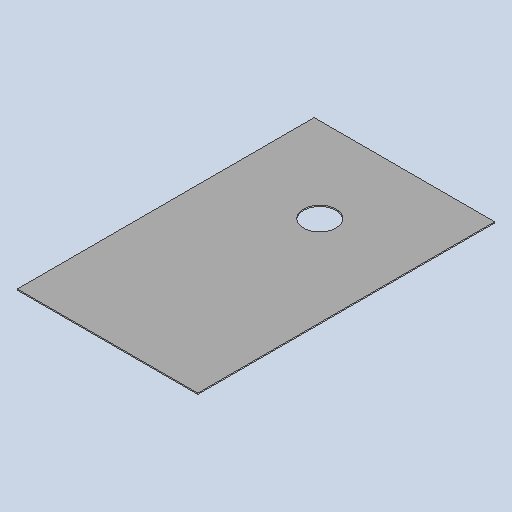
# Autodesk Inventor part: TRM 011 bottom main
Saved by Autodesk Inventor 2025 (Build 290162010, 162A)
## iProperties
Created: 2024-08-07
Part Number: TRM 011 bottom main
Material: AISI 304
Document SubType Name: Sheet Metal
Designer: pokla
Density: 8.02768 g/cm^3
Flat Pattern Width: 80.6 cm
Flat Pattern Length: 49 cm
Flat Pattern Area: 3949.4 cm^2
Sheet Metal Rule: AISI304 2mm Die16
Sheet Metal Width: 806.000 mm
Sheet Metal Length: 490.000 mm
Sheet Metal Area: 394940.000 mm^2
Appearance: Default
Stock Number: ТРМ 011 дно основное
Mass: 9361.53 g
Surface Area: 7860.53 cm^2
Volume: 1166.16 cm^3
Author: pokla
Autodesk Inventor part; units mm, degrees
ref_plane "YZ Plane" through (0, 0, 0) normal (1, 0, 0) x (0, 1, 0)
ref_plane "XZ Plane" through (0, 0, 0) normal (0, 1, 0) x (-1, 0, 0)
ref_plane "XY Plane" through (0, 0, 0) normal (0, 0, 1) x (1, 0, 0)
sketch "Sketch1" plane through (0, 0, 0) normal (0, 0, 1) x (1, 0, 0)
  line L0 (-245, -403) -> (245, -403)
  line L1 (245, -403) -> (245, 403)
  line L2 (245, 403) -> (-245, 403)
  line L3 (-245, 403) -> (-245, -403)
  line L4 (-245, -403) -> (245, 403) construction
  line L5 (245, -403) -> (-245, 403) construction
  point P0 (0, 0)
  dimension "d0" = 490
  dimension "d1" = 806
  measures "d0" distance of L2.end L1.end
  measures "d1" distance of L1.end L0.end
extrude "Plate1" add sketch "Sketch1" along normal blind 3
sketch "Sketch2" plane through (0, 0, 0) normal (0, 0, -1) x (-1, 0, 0)
  line L0 (-245, 403) -> (245, 403) projected
  line L1 (-245, -403) -> (-245, 403) projected
  line L2 (-225, 383) -> (-25, 383) construction
  line L3 (-25, 383) -> (-25, 363) construction
  line L4 (-25, 363) -> (-225, 363) construction
  line L5 (-225, 363) -> (-225, 383) construction
  point P0 (0, 0)
  dimension "d8" = 200
  dimension "d9" = 20
  dimension "d10" = 20
  dimension "d11" = 20
  constraints: 2 other
  measures "d8" distance of L2.start L2.end
  measures "d9" distance of L2.end L3.end
  measures "d10" distance between parallel lines of L0 L2
  measures "d11" distance between parallel lines of L1 L5
mark "Mark3"
sketch "Sketch6" plane through (0, 0, 3) normal (0, 0, 1) x (1, 0, 0)
  circle A0 centre (0, 173.1375) radius 44.5
  point P0 (0, 0)
  dimension "d42" = 89
  constraints: 1 centre point
  measures "d42" diameter of A0
extrude "Cut1" cut sketch "Sketch6" against normal blind 3
equation "\"d43\" = Thickness"
equation "\"d2\" = Thickness"
equation "\"BendReliefWidth\" = Thickness"
equation "\"BendReliefDepth\" = 0.5 * Thickness"
equation "\"CornerReliefSize\" = 4 * Thickness"
equation "\"MinimumRemnant\" = 2 * Thickness"
equation "\"TransitionRadius\" = BendRadius"
equation "\"JacobiRadiusSize\" = BendRadius"
equation "\"GapSize\" = Thickness"
equation "\"Thickness\" = 3"
equation "\"BendRadius\" = 2.75"
body "Solid1"
